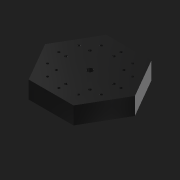
# Autodesk Inventor part: Spur Gear1
Saved by Autodesk Inventor 2017 (Build 210142000, 142)
## iProperties
Created: 2019-08-28
Part Number: Spur Gear1
Material: ABS Plastic
Document SubType Name: Modeling
Designer: Dell
Categories: <?xml version="1.0" encoding="UTF-16"?> <MemberInstance><Categories><FamilyTemplate><FamilyTemplateParameter ValueType="xs:double" Id="1" ObjectReferenceKey="da_z" ObjectType="kUserParameterObject"/><FamilyTemplateParameter ValueType="xs:double" Id="2" ObjectReferenceKey="da_b" ObjectType="kUserParameterObject"/><FamilyTemplateParameter ValueType="xs:double" Id="3" ObjectReferenceKey="da_beta" ObjectType="kUserParameterObject"/><FamilyTemplateParameter ValueType="xs:double" Id="4" ObjectReferenceKey="da_da" ObjectType="kUserParameterObject"/><FamilyTemplateParameter ValueType="xs:double" Id="5" ObjectReferenceKey="da_aw" ObjectType="kUserParameterObject"/><FamilyTemplateParameter ValueType="xs:string" Id="6" ObjectReferenceKey="EAIAABAAAACIAQAAAAAAAIAAAAAAAAAA" ObjectType="83910656" SubObjectId="SurfaceGeometry"/></FamilyTemplate><ParamToTemplateMap><ParamToTemplate CategoryParameter="//CategoryParameter[@InternalName='046C89C9-8512-4d59-83FE-43B91F4F132A']" TemplateParameter="1"/><ParamToTemplate CategoryParameter="//CategoryParameter[@InternalName='2552DF32-E462-4b46-AEBF-C6C7768E72AC']" TemplateParameter="2"/><ParamToTemplate CategoryParameter="//CategoryParameter[@InternalName='C9EE641D-15FC-4fae-A226-E94C4372FDD7']" TemplateParameter="3"/><ParamToTemplate><ParamToTemplate CategoryParameter="//CategoryParameter[@InternalName='00B6519A-459B-49c7-AD84-2E56D39A5744']" ConstantValue="0.000000"/></ParamToTemplate><ParamToTemplate><ParamToTemplate CategoryParameter="//CategoryParameter[@InternalName='04B31F0E-C7A6-4894-AA32-9629BEFACF47']" ConstantValue="1.000000"/></ParamToTemplate><ParamToTemplate><ParamToTemplate CategoryParameter="//CategoryParameter[@InternalName='43CBEC2E-7847-49e7-A936-2F7889FCB2D9']" ConstantValue="0.250000"/></ParamToTemplate><ParamToTemplate><ParamToTemplate CategoryParameter="//CategoryParameter[@InternalName='B1EFC894-105D-4ebd-86BF-FA20ED196853']" ConstantValue="0.350000"/></ParamToTemplate><ParamToTemplate><ParamToTemplate CategoryParameter="//CategoryParameter[@InternalName='51175063-3D10-4879-93E8-6246FE8B403D']" ConstantValue="2060000000.000000"/></ParamToTemplate><ParamToTemplate><ParamToTemplate CategoryParameter="//CategoryParameter[@InternalName='A3A52E27-4454-46a9-B0BD-C932399B70AF']" ConstantValue="0.300000"/></ParamToTemplate><ParamToTemplate><ParamToTemplate CategoryParameter="//CategoryParameter[@InternalName='91B76062-C214-41d9-B1B9-14D2AB99603D']" ConstantValue="0.200000"/></ParamToTemplate><ParamToTemplate><ParamToTemplate CategoryParameter="//CategoryParameter[@InternalName='374E806E-8B8A-4dda-A9AA-1039D6500AD2']" ConstantValue="5.000000"/></ParamToTemplate><ParamToTemplate><ParamToTemplate CategoryParameter="//CategoryParameter[@InternalName='2D373A89-B862-43d6-8D0B-0CBF12AB9F6C']" ConstantValue="0.392699"/></ParamToTemplate><ParamToTemplate CategoryParameter="//CategoryParameter[@InternalName='37777632-D6A2-4fac-9D53-DB8ACD95C989']" TemplateParameter="4"/><ParamToTemplate CategoryParameter="//CategoryParameter[@InternalName='FD1017F1-B727-4f7e-9707-0F86F1FF9423']" TemplateParameter="5"/><ParamToTemplate><ParamToTemplate CategoryParameter="//CategoryParameter[@InternalName='9E1B4470-B2D3-4ff1-B813-535BB4CDF51A']" ConstantValue="3520000.000000"/></ParamToTemplate><ParamToTemplate><ParamToTemplate CategoryParameter="//CategoryParameter[@InternalName='F8452263-BFF6-458c-9FB1-07C4B99E95CD']" ConstantValue="11400000.000000"/></ParamToTemplate><ParamToTemplate><ParamToTemplate CategoryParameter="//CategoryParameter[@InternalName='3E3BB259-FD49-497f-8171-6EBC954A3479']" ConstantValue="2.000000"/></ParamToTemplate><ParamToTemplate CategoryParameter="//CategoryParameter[@InternalName='27C3BAF2-7550-4e4b-AE2C-0DB134B7D9B7']" TemplateParameter="6"/></ParamToTemplateMap><Category DisplayName="Gear" InternalName="DC85795E-93AB-48d5-8EEE-5A27447B64BD" Mnemonic="Gear"><CategoryParameter DisplayName="z" InternalName="046C89C9-8512-4d59-83FE-43B91F4F132A" Mnemonic="z"/><CategoryParameter DisplayName="b" InternalName="2552DF32-E462-4b46-AEBF-C6C7768E72AC" Mnemonic="b"/><CategoryParameter DisplayName="||b|" InternalName="C9EE641D-15FC-4fae-A226-E94C4372FDD7" Mnemonic="beta"/><CategoryParameter DisplayName="x" InternalName="00B6519A-459B-49c7-AD84-2E56D39A5744" Mnemonic="x"/><CategoryParameter DisplayName="a*" InternalName="04B31F0E-C7A6-4894-AA32-9629BEFACF47" Mnemonic="a"/><CategoryParameter DisplayName="c*" InternalName="43CBEC2E-7847-49e7-A936-2F7889FCB2D9" Mnemonic="c"/><CategoryParameter DisplayName="r|.f|*" InternalName="B1EFC894-105D-4ebd-86BF-FA20ED196853" Mnemonic="rf"/><CategoryParameter DisplayName="E" InternalName="51175063-3D10-4879-93E8-6246FE8B403D" Mnemonic="E"/><CategoryParameter DisplayName="||m|" InternalName="A3A52E27-4454-46a9-B0BD-C932399B70AF" Mnemonic="mi"/><Category DisplayName="SpurGear" InternalName="26C5A22E-A91E-4dfd-A3B3-23CCAFAE1764" Mnemonic="SpurGear"><CategoryParameter DisplayName="m" InternalName="91B76062-C214-41d9-B1B9-14D2AB99603D" Mnemonic="m"/><CategoryParameter DisplayName="P" InternalName="374E806E-8B8A-4dda-A9AA-1039D6500AD2" Mnemonic="PP"/><CategoryParameter DisplayName="||a|" InternalName="2D373A89-B862-43d6-8D0B-0CBF12AB9F6C" Mnemonic="alpha"/><CategoryParameter DisplayName="d|.a|" InternalName="37777632-D6A2-4fac-9D53-DB8ACD95C989" Mnemonic="da"/><CategoryParameter DisplayName="a|.w|" InternalName="FD1017F1-B727-4f7e-9707-0F86F1FF9423" Mnemonic="aw"/><CategoryParameter DisplayName="||s||.Flim|" InternalName="9E1B4470-B2D3-4ff1-B813-535BB4CDF51A" Mnemonic="sFlim"/><CategoryParameter DisplayName="||s||.Hlim|" InternalName="F8452263-BFF6-458c-9FB1-07C4B99E95CD" Mnemonic="sHlim"/><CategoryParameter DisplayName="type" InternalName="3E3BB259-FD49-497f-8171-6EBC954A3479" Mnemonic="type"/><CategoryParameter DisplayName="PitchDiameter" InternalName="27C3BAF2-7550-4e4b-AE2C-0DB134B7D9B7" Mnemonic="IDS_PITCHDIAM"/></Category></Category></Categories></MemberInstance>
Density: 1.06 g/cm^3
Appearance: Smooth - Black
CustomPartVersion: 1
Author: Dell
Autodesk Inventor part; units mm, degrees
sketch "Sketch1" plane through (0, 0, 0) normal (0, 0, 1) x (1, 0, 0)
  circle A0 centre (0, 0) radius 16
  dimension "d0" = 32
  constraints: 1 centre point
  measures "d0" diameter of A0
extrude "Extrusion1" add sketch "Sketch1" along normal blind 20
ref_plane "Work Plane2" through (0, 0, 10) normal (0, 0, 1) x (1, 0, 0)
sketch "Sketch2" plane through (0, 0, 0) normal (0, 0, -1) x (-1, 0, 0)
  circle A0 centre (0, 0) radius 16 projected
  circle A1 centre (0, 0) radius 14
  dimension "d3" = 28
  constraints: 1 centre point, 1 coincident
  measures "d3" diameter of A1
surface extrude "Pitch Diameter" sketch "Sketch2" against normal through all shown no curves A1
ref_plane "Work Plane8" through (0, 0, 0) normal (0.9749279, 0.2225209, 0) x (0, 0, 1)
ref_plane "Work Plane9" through (0, 0, 0) normal (1, 0, 0) x (0, 1, 0)
spur gear teeth "Spur Gear" teeth 14 pitch diameter 28 tip diameter 32 root diameter 23 face width 20 start plane through (0, 0, 0) normal (0, 0, -1) x (-1, 0, 0)
sketch "Sketch4" plane through (0, 0, 0) normal (0, 0, -1) x (-1, 0, 0)
  circle A0 centre (0, 0) radius 4.7625
  dimension "d53" = 9.525
  constraints: 1 centre point, 1 coincident
  measures "d53" diameter of A0
extrude "Extrusion3" cut sketch "Sketch4" against normal through all
sketch "Sketch5" plane through (0, 0, 20) normal (0, 0, 1) x (1, 0, 0)
  circle A0 centre (0, 0) radius 17
  circle A1 centre (0, 0) radius 4.7625 projected
  dimension "d56" = 34
  constraints: 1 centre point, 1 coincident
  measures "d56" diameter of A0
extrude "Extrusion4" add sketch "Sketch5" along normal blind 28
sketch "Sketch8" plane through (0, 0, 48) normal (0, 0, 1) x (1, 0, 0)
  circle A0 centre (0, 0) radius 4.7625 projected
  circle A1 centre (0, 0) radius 17 projected
  circle A2 centre (0, 0) radius 67.5
  circle A3 centre (0, 41.5) radius 2.25
  circle A4 centre (-29.3449, 29.3449) radius 2.25
  circle A5 centre (-41.5, 0) radius 2.25
  circle A6 centre (-29.3449, -29.3449) radius 2.25
  circle A7 centre (0, -41.5) radius 2.25
  circle A8 centre (29.3449, -29.3449) radius 2.25
  circle A9 centre (41.5, 0) radius 2.25
  circle A10 centre (29.3449, 29.3449) radius 2.25
  dimension "d59" = 135
  dimension "d60" = 4.5
  dimension "d61" = 41.5
  dimension "d64" = 360
  constraints: 9 centre point, 1 coincident, 1 vertical alignment, 17 other
  measures "d59" diameter of A2
  measures "d60" diameter of A3
  measures "d61" distance of point (0, 0) A3.centre
extrude "Extrusion5" add sketch "Sketch8" along normal blind 10 contours A1 | A2
sketch "Sketch9" plane through (0, 0, 48) normal (0, 0, -1) x (-1, 0, 0)
  circle A0 centre (0, 0) radius 33
  circle A1 centre (0, 0) radius 67.5 projected
  circle A2 centre (0, 41.5) radius 2.25 projected
  circle A3 centre (29.3449, 29.3449) radius 2.25 projected
  circle A4 centre (41.5, 0) radius 2.25 projected
  circle A5 centre (29.3449, -29.3449) radius 2.25 projected
  circle A6 centre (0, -41.5) radius 2.25 projected
  circle A7 centre (0, -41.5) radius 2.25 projected
  circle A8 centre (-29.3449, -29.3449) radius 2.25 projected
  circle A9 centre (-29.3449, -29.3449) radius 2.25 projected
  circle A10 centre (-29.3449, 29.3449) radius 2.25 projected
  circle A11 centre (-29.3449, 29.3449) radius 2.25 projected
  circle A12 centre (-41.5, 0) radius 2.25 projected
  circle A13 centre (-41.5, 0) radius 2.25 projected
  dimension "d68" = 66
  constraints: 1 centre point, 1 coincident
  measures "d68" diameter of A0
extrude "Extrusion6" add sketch "Sketch9" along normal blind 3
sketch "Sketch11" plane through (0, 0, 45) normal (0, 0, -1) x (-1, 0, 0)
  circle A0 centre (0, 0) radius 48
  circle A1 centre (0, 0) radius 67.5 projected
  dimension "d73" = 96
  constraints: 1 centre point, 1 coincident
  measures "d73" diameter of A0
extrude "Extrusion8" add sketch "Sketch11" along normal blind 15
sketch "Sketch12" plane through (0, 0, 58) normal (0, 0, 1) x (1, 0, 0)
  circle A0 centre (0, -54) radius 2
  circle A1 centre (27, -46.7654) radius 2
  circle A2 centre (46.7654, -27) radius 2
  circle A3 centre (54, 0) radius 2
  circle A4 centre (46.7654, 27) radius 2
  circle A5 centre (27, 46.7654) radius 2
  circle A6 centre (0, 54) radius 2
  circle A7 centre (-27, 46.7654) radius 2
  circle A8 centre (-46.7654, 27) radius 2
  circle A9 centre (-54, 0) radius 2
  circle A10 centre (-46.7654, -27) radius 2
  circle A11 centre (-27, -46.7654) radius 2
  point P0 (0, 0)
  dimension "d76" = 4
  dimension "d77" = 54
  dimension "d80" = 360
  constraints: 12 centre point, 1 vertical alignment, 25 other
  measures "d76" diameter of A0
  measures "d77" distance of A0.centre point (0, 0)
extrude "Extrusion9" cut sketch "Sketch12" against normal through all
sketch "Sketch15" plane through (0, 0, 30) normal (0, 0, -1) x (-1, 0, 0)
  line L0 (77.9423, 0) -> (38.9711, -67.5)
  line L1 (38.9711, -67.5) -> (-38.9711, -67.5)
  line L2 (-38.9711, -67.5) -> (-77.9423, 0)
  line L3 (-77.9423, 0) -> (-38.9711, 67.5)
  line L4 (-38.9711, 67.5) -> (38.9711, 67.5)
  line L5 (38.9711, 67.5) -> (77.9423, 0)
  circle A0 centre (0, 0) radius 67.5 projected
  constraints: 12 end point, 1 coincident, 1 horizontal alignment, 1 tangent, 13 other
extrude "Extrusion10" add sketch "Sketch15" against normal blind 28 contours L0 A0 L5 | L0 L1 A0 | A0 L4 L5 | L1 L2 A0 | A0 L3 L4 | L2 L3 A0
sketch "Sketch16" plane through (0, 0, 58) normal (0, 0, 1) x (1, 0, 0)
  circle A0 centre (-46.7654, -27) radius 2 projected
  circle A1 centre (-46.7654, 27) radius 2 projected
  circle A2 centre (0, 54) radius 2 projected
  circle A3 centre (46.7654, 27) radius 2 projected
  circle A4 centre (46.7654, -27) radius 2 projected
  circle A5 centre (0, -54) radius 2 projected
  circle A6 centre (27, -46.7654) radius 2 projected
  circle A7 centre (54, 0) radius 2 projected
  circle A8 centre (27, 46.7654) radius 2 projected
  circle A9 centre (-27, 46.7654) radius 2 projected
  circle A10 centre (-54, 0) radius 2 projected
  circle A11 centre (-27, -46.7654) radius 2 projected
  circle A12 centre (0, 0) radius 4.7625 projected
  circle A13 centre (29.3449, 29.3449) radius 2.25 projected
  circle A14 centre (41.5, 0) radius 2.25 projected
  circle A15 centre (29.3449, -29.3449) radius 2.25 projected
  circle A16 centre (0, -41.5) radius 2.25 projected
  circle A17 centre (-29.3449, -29.3449) radius 2.25 projected
  circle A18 centre (-41.5, 0) radius 2.25 projected
  circle A19 centre (-29.3449, 29.3449) radius 2.25 projected
  circle A20 centre (0, 41.5) radius 2.25 projected
  line L0 (77.9423, 0) -> (38.9711, 67.5) projected
  line L1 (38.9711, 67.5) -> (-38.9711, 67.5) projected
  line L2 (-38.9711, 67.5) -> (-77.9423, 0) projected
  line L3 (-77.9423, 0) -> (-38.9711, -67.5) projected
  line L4 (-38.9711, -67.5) -> (38.9711, -67.5) projected
  line L5 (38.9711, -67.5) -> (77.9423, 0) projected
extrude "Extrusion11" add sketch "Sketch16" along normal blind 2
equation "\"d0\" = da_da"
equation "\"d1\" = da_b"
equation "\"d3\" = da_dw"
equation "\"d16\" = da_aw"
equation "\"d43\" = da_aw"
equation "\"d46\" = da_aw"
equation "\"da_da\" = 32"
equation "\"da_b\" = 20"
equation "\"da_dw\" = 28"
equation "\"da_aw\" = 28"
body "Solid1"
body "Srf1"
